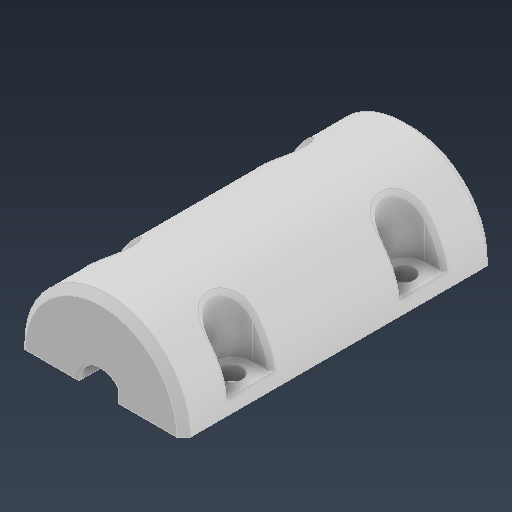
# Autodesk Inventor part: stepperToAxleConnector_1
Saved by Autodesk Inventor 2021.4 (Build 254397000, 397)
## iProperties
Created: 2022-03-02
Part Number: stepperToAxleConnector_1
Material: Generic
Document SubType Name: Modeling
Designer: jo_ki
Density: 1 g/cm^3
Appearance: Default
Author: jo_ki
Autodesk Inventor part; units mm, degrees
ref_plane "YZ Plane" through (0, 0, 0) normal (1, 0, 0) x (0, 1, 0)
derived "Mastersketch.ipt"
sketch "Sketch3" plane through (0, 0, 0) normal (1, 0, 0) x (0, 1, 0)
  line L0 (3.175, 17.5) -> (5, 17.5)
  line L1 (5, 17.5) -> (5, 2.5)
  line L2 (5, 2.5) -> (3.175, 2.5)
  line L3 (3.175, 2.5) -> (3.175, 17.5)
  line L4 (5, 17.5) -> (12, 17.5)
  line L5 (12, 17.5) -> (12, -27.5)
  line L6 (12, -27.5) -> (5, -27.5)
  line L7 (5, -27.5) -> (5, 17.5)
  line L8 (0, -36.5) -> (0, 26.5) projected
  point P0 (0, 0)
  dimension "d1" = 10
  dimension "d3" = 6.35
  dimension "d7" = 7
  dimension "d8" = 30
  dimension "d9" = 15
  dimension "d10" = 2.5
  constraints: 16 end point, 4 parallel, 2 horizontal, 2 perpendicular
  measures "d1" diameter of L7 L8
  measures "d3" diameter of L3 L8
  measures "d7" distance between parallel lines of L7 L5
  measures "d8" distance between parallel lines of L2 L6
  measures "d9" distance between parallel lines of L0 L2
  measures "d10" distance from line of point (0, 0) L2
revolve "Revolution1" add sketch "Sketch3" angle 180 mid plane about axis through (0, 0, -10) along (0, 0, 1)
chamfer "Chamfer1" distance 1 angle 45 2 edges at (0, 12, -27.5) (0, 12, 17.5)
sketch "Sketch4" plane through (0, 0, 0) normal (0, 1, 0) x (-1, 0, 0)
  line L0 (-11, 17.5) -> (-3.175, 17.5) projected
  line L1 (3.175, 2.5) -> (-3.175, 2.5) projected
  line L2 (-3.175, 17.5) -> (-2.625, 17.5)
  line L3 (-2.625, 17.5) -> (-2.625, 2.5)
  line L4 (-2.625, 2.5) -> (-3.175, 2.5)
  line L5 (-3.175, 2.5) -> (-3.175, 17.5)
  line L6 (-3.175, 2.5) -> (-5, 2.5) projected
  line L7 (11, -27.5) -> (-11, -27.5) projected
  line L8 (-5, 2.5) -> (-3, 2.5)
  line L9 (-3, 2.5) -> (-3, -27.5)
  line L10 (-3, -27.5) -> (-5, -27.5)
  line L11 (-5, -27.5) -> (-5, 2.5)
  point P0 (0, 0)
  dimension "d19" = 2
  dimension "d20" = 0.55
  constraints: 16 end point, 4 parallel, 2 horizontal, 2 perpendicular, 2 point on line
  measures "d19" distance between parallel lines of L9 L11
  measures "d20" distance between parallel lines of L5 L3
extrude "Extrusion1" add sketch "Sketch4" along normal up to surface round surface about axis through (0, 0, -12.5) along (0, 0, 1) radius 5 far side no
sketch "Sketch6" plane through (0, 0, 0) normal (0, 1, 0) x (-1, 0, 0)
  line L0 (12, -20.5) -> (6, -20.5)
  line L1 (6, -20.5) -> (6, -14.5)
  line L2 (6, -14.5) -> (12, -14.5)
  line L3 (12, -14.5) -> (12, -20.5)
  line L4 (12, 16.5) -> (12, -26.5) projected
  line L5 (11, -27.5) -> (5, -27.5) projected
  circle A0 centre (9, -17.5) radius 3
  circle A1 centre (9, -17.5) radius 1.5
  point P0 (0, 0)
  point P1 (9, -14.5)
  point P2 (9, -20.5)
  dimension "d46" = 6
  dimension "d47" = 7
  dimension "d68" = 3
  constraints: 8 end point, 3 tangent, 2 centre point, 2 parallel, 2 perpendicular, 1 coincident, 1 collinear, 1 horizontal
  measures "d46" distance between parallel lines of L3 L1
  measures "d47" distance between parallel lines of L0 L5
  measures "d68" diameter of A1
ref_plane "Work Plane1" through (0, 2, 0) normal (0, 1, 0) x (-1, 0, 0)
extrude "Extrusion3" cut sketch "Sketch6" along normal blind 10 from surface at 2 contours L0 A0 L3 | A0 | A0 L2 L3 | A1
extrude "Extrusion4" cut sketch "Sketch6" along normal blind 2 contours A1
chamfer "Chamfer2" distance 0.5 angle 45 3 edges at (-6, 10.3923, -17.4999) (-10.8309, 5.1665, -14.5) (-10.8309, 5.1665, -20.5)
ref_plane "Work Plane2" through (0, 0, -5) normal (0, 0, -1) x (-1, 0, 0)
mirror "Mirror1" about plane through (0, 0, -5) normal (0, 0, -1) of "Extrusion3", "Chamfer2", "Extrusion4"
mirror "Mirror2" about plane through (0, 0, 0) normal (1, 0, 0) of "Extrusion3", "Mirror1", "Chamfer2", "Extrusion4"
body "Solid1"
